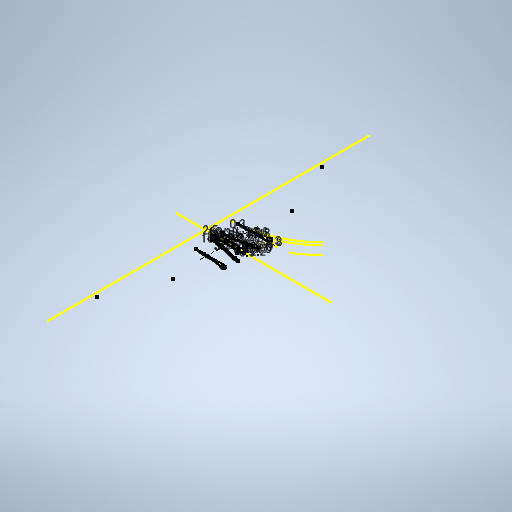
# Autodesk Inventor part: RR_SingleTurnoutLever-ALL
Saved by Autodesk Inventor 2025.1 (Build 291241000, 241)
## iProperties
Created: 2025-03-06
Part Number: RR_SingleTurnoutLever-ALL
Material: 一般
Document SubType Name: Modeling
Designer: kumagai
Density: 1 g/cm^3
Appearance: 既定
Author: kumagai
Autodesk Inventor part; units mm, degrees
ref_plane "YZ Plane" through (0, 0, 0) normal (1, 0, 0) x (0, 1, 0)
ref_plane "XZ Plane" through (0, 0, 0) normal (0, 1, 0) x (-1, 0, 0)
ref_plane "XY Plane" through (0, 0, 0) normal (0, 0, 1) x (1, 0, 0)
derived "RR_ThreeWay.ipt"
sketch "MainSketch" plane through (0, 0, 0) normal (0, 1, 0) x (-1, 0, 0)
  line L0 (0, -344.2613) -> (0, 286.2613)
  line L1 (-272.9287, 0) -> (62.5724, 0)
  line L2 (14.6437, -29) -> (-5, -29)
  line L3 (-5, -49.5106) -> (-5, -5.6416)
  line L4 (-5, -48) -> (0, -48)
  line L5 (-5, -10) -> (0, -10)
  line L6 (-5, -38.3) -> (0, -38.3)
  line L7 (-5, -19.7) -> (0, -19.7)
  line L8 (-5, -46) -> (0, -46)
  line L9 (-5, -35.9) -> (0, -35.9)
  line L10 (-5, -22.1) -> (0, -22.1)
  line L11 (-5, -12) -> (0, -12)
  line L12 (-10, -10) -> (-10, -29)
  line L13 (-225, -48) -> (-225, -29)
  line L14 (-120.9077, -19.7) -> (-225, -19.7)
  arc A0 (-10, -48) -> (-148.5929, -105.4071) centre (-10, -244) ccw
  arc A1 (-10, -46) -> (-150.0071, -103.9929) centre (-10, -244) ccw
  line L15 (-143.2215, -110.7785) -> (-189.5102, -64.4898)
  line L16 (-210, -35.9) -> (-210, -29)
  line L17 (-146.1596, -86.6272) -> (-155.9415, -76.8453)
  arc A2 (-133.8847, -47.8455) -> (-174.0488, -79.9512) centre (-10, -244) ccw
  arc A3 (-139.2229, -48.9168) -> (-175.463, -78.537) centre (-10, -244) ccw
  line L18 (-139.499, -48) -> (-225, -48)
  line L19 (-134.4186, -46) -> (-225, -46)
  arc A4 (-118.9103, -50.6657) -> (-166.907, -87.093) centre (-10, -244) ccw
  arc A5 (-120.0882, -48.5746) -> (-168.6041, -85.3959) centre (-10, -244) ccw
  line L20 (-94.2219, -46) -> (-110.2721, -46)
  arc A6 (-111.9271, -35.5897) -> (-114.1724, -36.7028) centre (-10, -244) ccw
  line L21 (-120.9077, -35.9) -> (-225, -35.9)
  line L22 (-120.9077, -38.3) -> (-225, -38.3)
  arc A7 (-133.8847, -47.8455) -> (-134.4186, -46) centre (-134.4186, -47) ccw
  arc A8 (-139.2229, -48.9168) -> (-139.499, -48) centre (-139.499, -48.5) ccw
  arc A9 (-110.2721, -48.4) -> (-118.9103, -50.6657) centre (-110.2721, -66) ccw
  arc A10 (-110.2721, -46) -> (-120.0882, -48.5746) centre (-110.2721, -66) ccw
  arc A11 (-120.9077, -38.3) -> (-114.1724, -36.7028) centre (-120.9077, -23.3) ccw
  arc A12 (-120.9077, -35.9) -> (-115.25, -34.5584) centre (-120.9077, -23.3) ccw
  arc A13 (-143.5264, -51.2283) -> (-148.5252, -54.7884) centre (-10, -244) ccw
  arc A14 (-112.9815, -33.4337) -> (-115.25, -34.5584) centre (-10, -244) ccw
  line L23 (-120.9077, -22.1) -> (-225, -22.1)
  circle A15 centre (-86.125, -22.2) radius 2.5
  arc A16 (-96.415, -52.9331) -> (-105.3417, -57.2273) centre (-10, -244) ccw
  arc A17 (-96.4922, -49.4759) -> (-95.7188, -53.2122) centre (-89.6121, -50) ccw
  arc A18 (-93.3838, -47.5455) -> (-92.1285, -53.7307) centre (-89.6121, -50) ccw
  arc A19 (-96.1897, -54.5879) -> (-157.1489, -96.8511) centre (-10, -244) ccw
  line L24 (-97.4893, -48.4) -> (-110.2721, -48.4)
  arc A20 (-92.2877, -55.4762) -> (-155.4519, -98.5481) centre (-10, -244) ccw
  arc A21 (-92.2877, -55.4762) -> (-92.1285, -53.7307) centre (-92.6877, -54.5597) ccw
  arc A22 (-93.3838, -47.5455) -> (-94.2219, -46) centre (-94.2219, -47) ccw
  arc A23 (-96.1897, -54.5879) -> (-95.7188, -53.2122) centre (-96.6039, -53.6777) ccw
  arc A24 (-96.4922, -49.4759) -> (-97.4893, -48.4) centre (-97.4893, -49.4) ccw
  circle A25 centre (-89.6121, -50) radius 2.5
  line L25 (-42.4799, -17.7596) -> (-25.8571, -19.9879)
  arc A26 (-25.9153, -20.5847) -> (-85.6348, -24.6515) centre (-40.1446, -252.1479) ccw
  arc A27 (-85.7928, -19.7222) -> (-85.6348, -24.6515) centre (-86.125, -22.2) ccw
  arc A28 (-25.9153, -20.5847) -> (-25.8571, -19.9879) centre (-25.8969, -20.2853) ccw
  arc A29 (-42.4799, -17.7596) -> (-76.3848, -20.5664) centre (-40.1446, -252.1479) ccw
  line L26 (-85.7928, -19.7222) -> (-79.2595, -20.598)
  arc A30 (-79.2595, -20.598) -> (-76.3848, -20.5664) centre (-77.9308, -10.6866) ccw
  circle A31 centre (-89.6121, -50) radius 4
  line L27 (-89.754, -46.0025) -> (-25.5965, -43.7259)
  arc A32 (-25.552, -44.3238) -> (-40.8225, -46.6677) centre (-3.1703, -241.0547) ccw
  arc A33 (-25.552, -44.3238) -> (-25.5965, -43.7259) centre (-25.5859, -44.0257) ccw
  arc A34 (-74.4895, -48.1141) -> (-87.9633, -53.6443) centre (-3.1703, -241.0547) ccw
  line L28 (-72.9332, -47.8071) -> (-40.8225, -46.6677)
  arc A35 (-72.9332, -47.8071) -> (-74.4895, -48.1141) centre (-72.7559, -52.804) ccw
  arc A36 (-44.0479, -18.9806) -> (-84.6326, -23.2308) centre (-40.1446, -252.1479) ccw
  arc A37 (-27.9859, -39.0878) -> (-44.4613, -41.2072) centre (-10, -244) ccw
  line L29 (-31.1334, -19.7) -> (-47.6548, -19.7)
  arc A38 (-10, -22.1) -> (-22.0271, -22.4262) centre (-10, -244) ccw
  arc A39 (-44.7432, -24.8368) -> (-62.9678, -28.5145) centre (-10, -244) ccw
  arc A40 (-10, -19.7) -> (-22.1572, -20.0297) centre (-10, -244) ccw
  arc A41 (-45.119, -22.4664) -> (-72.2793, -28.5197) centre (-10, -244) ccw
  arc A42 (-25.457, -23.6967) -> (-43.178, -22.3501) centre (-51.8841, -254.1867) ccw
  line L30 (-24.9, -22.9254) -> (-24.9, -23.2)
  arc A43 (-25.457, -23.6967) -> (-24.9, -23.2) centre (-25.4, -23.2) ccw
  arc A44 (-22.1572, -20.0297) -> (-24.9, -22.9254) centre (-22, -22.9254) ccw
  arc A45 (-43.178, -22.3501) -> (-45.119, -22.4664) centre (-43.5532, -32.343) ccw
  arc A46 (-25.7303, -26.0811) -> (-43.268, -24.7484) centre (-51.8841, -254.1867) ccw
  arc A47 (-22.0271, -22.4262) -> (-22.5, -22.9254) centre (-22, -22.9254) ccw
  line L31 (-22.5, -22.9254) -> (-22.5, -23.2)
  arc A48 (-25.7303, -26.0811) -> (-22.5, -23.2) centre (-25.4, -23.2) ccw
  arc A49 (-43.268, -24.7484) -> (-44.7432, -24.8368) centre (-43.5532, -32.343) ccw
  line L32 (-55.2, -53.283) -> (-55.2, -10)
  line L33 (-40.8, -50.4351) -> (-40.8, -10)
  line L34 (-48, 3.552) -> (-48, 5.2256)
  line L35 (-59, -61.5) -> (-37, -61.5)
  line L36 (-40.8, -10) -> (-40.8, -7.4996)
  line L37 (-55.2, -10) -> (-55.2, -7.4996)
  line L38 (-48, -61.9179) -> (-48, -64.1825)
  line L39 (-37, -61.5) -> (-37, -70.5)
  line L40 (-40, -73.5) -> (-42, -73.5)
  line L41 (-42, -73.5) -> (-40, -62)
  line L42 (-40, -62) -> (-56, -62)
  line L43 (-56, -62) -> (-54, -73.5)
  line L44 (-54, -73.5) -> (-56, -73.5)
  line L45 (-59, -70.5) -> (-59, -58.1371)
  arc A50 (-40, -73.5) -> (-37, -70.5) centre (-40, -70.5) ccw
  arc A51 (-59, -70.5) -> (-56, -73.5) centre (-56, -70.5) ccw
  line L46 (-37, -61.5) -> (-37, -49.8686)
  line L47 (-40.8, -50.4351) -> (-40.8, -62)
  line L48 (-55.2, -53.283) -> (-55.2, -62)
  arc A52 (-34.3731, -49.5213) -> (-37, -52.498) centre (-34, -52.498) ccw
  arc A53 (-59, -58.1371) -> (-62.8083, -55.2481) centre (-62, -58.1371) ccw
  line L49 (-10, -29) -> (-225, -29)
  arc A54 (-151.7465, 120.5538) -> (-11.4945, 29.8813) centre (-10, 186) ccw
  arc A55 (-22.0271, -35.5738) -> (-10, -35.9) centre (-10, 186) ccw
  arc A56 (-22.1572, -37.9703) -> (-10, -38.3) centre (-10, 186) ccw
  arc A57 (-43.268, -33.2516) -> (-25.7303, -31.9189) centre (-51.8841, 196.1867) ccw
  arc A58 (-43.178, -35.6499) -> (-25.457, -34.3033) centre (-51.8841, 196.1867) ccw
  arc A59 (-62.9678, -29.4855) -> (-44.7432, -33.1632) centre (-10, 186) ccw
  arc A60 (-72.2793, -29.4803) -> (-45.119, -35.5336) centre (-10, 186) ccw
  arc A61 (-45.119, -35.5336) -> (-43.178, -35.6499) centre (-43.5532, -25.657) ccw
  arc A62 (-44.7432, -33.1632) -> (-43.268, -33.2516) centre (-43.5532, -25.657) ccw
  arc A63 (-22.5, -35.0746) -> (-22.0271, -35.5738) centre (-22, -35.0746) ccw
  arc A64 (-24.9, -35.0746) -> (-22.1572, -37.9703) centre (-22, -35.0746) ccw
  line L50 (-24.9, -35.0746) -> (-24.9, -34.8)
  line L51 (-22.5, -35.0746) -> (-22.5, -34.8)
  arc A65 (-24.9, -34.8) -> (-25.457, -34.3033) centre (-25.4, -34.8) ccw
  arc A66 (-22.5, -34.8) -> (-25.7303, -31.9189) centre (-25.4, -34.8) ccw
  arc A67 (-62.9678, -28.5145) -> (-63.3485, -29) centre (-62.8485, -29) ccw
  arc A68 (-72.2793, -28.5197) -> (-72.6405, -29) centre (-72.1405, -29) ccw
  arc A69 (-108.1902, -15.666) -> (-89.3785, -23.7845) centre (-10, 186) ccw
  arc A70 (-91.0057, 5.3288) -> (-16.6975, -11.8867) centre (-10, 186) ccw
  arc A71 (-122.8924, 131.193) -> (-43.8763, 65.1658) centre (-10, 186) ccw
  arc A72 (-148.5252, -3.2116) -> (-143.5264, -6.7717) centre (-10, 186) ccw
  circle A73 centre (-86.125, -35.8) radius 2.5
  arc A74 (-85.7286, -33.3316) -> (-25.8975, -35.1189) centre (-48.9436, 195.7336) ccw
  line L52 (-25.8166, -35.7131) -> (-42.3424, -38.5735)
  arc A75 (-25.8166, -35.7131) -> (-25.8975, -35.1189) centre (-25.8677, -35.4174) ccw
  line L53 (-85.6986, -38.2634) -> (-79.2034, -37.1391)
  arc A76 (-76.3296, -37.0611) -> (-79.2034, -37.1391) centre (-77.4979, -46.9926) ccw
  arc A77 (-76.3296, -37.0611) -> (-42.3424, -38.5735) centre (-48.9436, 195.7336) ccw
  arc A78 (-49.1227, -37.4664) -> (-46.0444, -37.4484) centre (-48.9436, 195.7336) ccw
  line L54 (-86.4807, -38.2746) -> (-94.1197, -37.1765)
  arc A79 (-94.2268, -36.2144) -> (-94.1197, -37.1765) centre (-94.0486, -36.6816) ccw
  line L55 (-87.0159, -33.4641) -> (-94.2268, -36.2144)
  line L56 (-76.4926, -34.8148) -> (-77.6457, -34.6296)
  arc A80 (-96.055, -36.8647) -> (-107.6082, -42.0517) centre (-10, -244) ccw
  circle A81 centre (-89.6121, -8) radius 4
  line L57 (-89.6178, -12) -> (-25.42, -12.0915)
  arc A82 (-88.0883, -4.3016) -> (-74.4341, -9.37) centre (-9.7235, 185.8863) ccw
  arc A83 (-74.4341, -9.37) -> (-72.8683, -9.6239) centre (-72.8611, -4.6239) ccw
  line L58 (-72.8683, -9.6239) -> (-40.7373, -9.6697)
  arc A84 (-40.7373, -9.6697) -> (-25.3959, -11.4925) centre (-9.7235, 185.8863) ccw
  arc A85 (-25.42, -12.0915) -> (-25.3959, -11.4925) centre (-25.4196, -11.7915) ccw
  line L59 (-41.4, -73.5) -> (-41.4, -70.05)
  line L60 (-54.6, -73.5) -> (-54.6, -70.05)
  line L61 (-21.7393, -64.7371) -> (-21.7393, -55.7371)
  line L62 (-51.6, 5.7033) -> (-51.6, 3.6437)
  line L63 (-44.4, 6.6538) -> (-44.4, 3.6437)
  line L64 (-44.4, -63.9796) -> (-44.4, -61.3243)
  line L65 (-51.6, -63.5159) -> (-51.6, -61.3243)
  arc A86 (-106.8215, -31.0506) -> (-105.9722, -29) centre (-108.8722, -29) ccw
  arc A87 (-111.9271, -35.5897) -> (-109.9456, -34.1747) centre (-115.1782, -28.9421) ccw
  line L66 (-109.9456, -34.1747) -> (-106.8215, -31.0506)
  arc A88 (-112.9815, -33.4337) -> (-111.6427, -32.4776) centre (-115.1782, -28.9421) ccw
  arc A89 (-108.5186, -29.3536) -> (-108.3722, -29) centre (-108.8722, -29) ccw
  line L67 (-111.6427, -32.4776) -> (-108.5186, -29.3536)
  arc A90 (-63.3485, -29) -> (-62.9678, -29.4855) centre (-62.8485, -29) ccw
  arc A91 (-72.6405, -29) -> (-72.2793, -29.4803) centre (-72.1405, -29) ccw
  line L68 (-210, -29) -> (-210, -22.1)
  line L69 (-225, -29) -> (-225, -10)
  line L70 (-10, -29) -> (-10, -48)
  line L71 (-22.0231, -12) -> (-39.3668, -12)
  line L72 (-157.1489, -96.8511) -> (-146.5423, -86.2445)
  point P0 (0, 0)
  point P1 (-90.8602, -19.7)
  point P2 (-94.9346, -22.1)
  point P3 (-96.3241, -48.4)
  point P4 (-87.5506, -46)
  point P5 (-162.028, -91.972)
  point P6 (-44.0258, -45.5806)
  point P7 (-48, -2.9806)
  point P8 (-48, -61.5806)
  point P9 (-37, -73.5)
  point P10 (-59, -73.5)
  point P11 (-51.2642, -37.4549)
  point P12 (-51.1178, -10.8549)
  point P13 (-103.3722, -29)
  point P14 (-48, -53.4549)
sketch "LeverSketch" plane through (0, 0, 0) normal (0, 1, 0) x (-1, 0, 0)
  circle A0 centre (-89.6121, -50) radius 4
  circle A1 centre (-86.125, -22.2) radius 2.5
  arc A2 (-26.6638, -12.5992) -> (-85.3134, -24.5646) centre (-10, -244) ccw
  arc A3 (-26.6638, -12.5992) -> (-26.6853, -12) centre (-26.6853, -12.3) ccw
  arc A4 (-43.4568, -12) -> (-76.6882, -19.2867) centre (-10, -244) ccw
  line L0 (-43.4568, -12) -> (-26.6853, -12)
  line L1 (-86.125, -19.7) -> (-79.5332, -19.7)
  arc A5 (-52.0572, -14.6238) -> (-62.7445, -16.8431) centre (-10, -244) ccw
  arc A6 (-79.5332, -19.7) -> (-76.6882, -19.2867) centre (-79.5332, -9.7) ccw
  line L2 (-89.6121, -46) -> (-25.4143, -46)
  line L3 (-59.4552, -48.4) -> (-40.735, -48.4)
  arc A7 (-25.391, -46.5991) -> (-40.735, -48.4) centre (-10, -244) ccw
  arc A8 (-25.391, -46.5991) -> (-25.4143, -46) centre (-25.4143, -46.3) ccw
  line L4 (0, -353.824) -> (0, 343.6373) projected
  line L5 (-272.9287, 0) -> (62.5724, 0) projected
  circle A9 centre (-86.125, 22.2) radius 2.5
  arc A10 (-85.3134, 24.5646) -> (-26.6638, 12.5992) centre (-10, 244) ccw
  arc A11 (-26.6853, 12) -> (-26.6638, 12.5992) centre (-26.6853, 12.3) ccw
  arc A12 (-76.6882, 19.2867) -> (-43.4568, 12) centre (-10, 244) ccw
  line L6 (-43.4568, 12) -> (-26.6853, 12)
  line L7 (-86.125, 19.7) -> (-79.5332, 19.7)
  arc A13 (-76.6882, 19.2867) -> (-79.5332, 19.7) centre (-79.5332, 9.7) ccw
  circle A14 centre (-89.6121, 50) radius 4
  line L8 (-89.6121, 46) -> (-25.4143, 46)
  line L9 (-59.4552, 48.4) -> (-40.735, 48.4)
  arc A15 (-88.1761, 53.7333) -> (-59.4552, 48.4) centre (-59.4552, 128.4) ccw
  arc A16 (-40.735, 48.4) -> (-25.391, 46.5991) centre (-10, 244) ccw
  arc A17 (-25.4143, 46) -> (-25.391, 46.5991) centre (-25.4143, 46.3) ccw
  circle A18 centre (-86.125, -22.2) radius 1.1
  circle A19 centre (-89.6121, -50) radius 1.1
  circle A20 centre (-86.125, 22.2) radius 1.1
  circle A21 centre (-89.6121, 50) radius 1.1
  circle A22 centre (-89.6121, -50) radius 2.4
  circle A23 centre (-86.125, -22.2) radius 2.4
  circle A24 centre (-89.6121, -50) radius 1.65
  circle A25 centre (-86.125, -22.2) radius 1.65
  circle A26 centre (-52.0572, -14.6238) radius 1.6
  circle A27 centre (-51.1138, -47.2) radius 1.6
  circle A28 centre (-52.0572, -14.6238) radius 1.8
  circle A29 centre (-51.1138, -47.2) radius 1.8
  circle A30 centre (-52.0572, 14.6238) radius 1.65
  circle A31 centre (-52.0572, 14.6238) radius 1.85
  circle A32 centre (-51.1138, 47.2) radius 1.65
  circle A33 centre (-51.1138, 47.2) radius 1.85
  line L10 (-60, -5.0418) -> (-60, -4.3264)
  line L11 (-33.7, -3.5) -> (-86.7, -3.5)
  line L12 (-87.2, -3) -> (-87.2, 3)
  line L13 (-86.7, 3.5) -> (-34.7, 3.5)
  arc A34 (-48.1, -1) -> (-45.3, -1) centre (-46.7, -1) ccw
  arc A35 (-45.3, 1) -> (-48.1, 1) centre (-46.7, 1) ccw
  line L14 (-45.3, -1) -> (-45.3, 1)
  line L15 (-48.1, -1) -> (-48.1, 1)
  arc A36 (-74.7, -1) -> (-71.9, -1) centre (-73.3, -1) ccw
  arc A37 (-71.9, 1) -> (-74.7, 1) centre (-73.3, 1) ccw
  line L16 (-74.7, -1) -> (-74.7, 1)
  line L17 (-71.9, -1) -> (-71.9, 1)
  circle A38 centre (-21.2, 3.6) radius 1.6
  arc A39 (-86.7, 3.5) -> (-87.2, 3) centre (-86.7, 3) ccw
  arc A40 (-87.2, -3) -> (-86.7, -3.5) centre (-86.7, -3) ccw
  arc A41 (-59.4552, -48.4) -> (-88.1761, -53.7333) centre (-59.4552, -128.4) ccw
  arc A42 (-10, -46) -> (-150.0071, -103.9929) centre (-10, -244) ccw projected
  arc A43 (-92.2877, -55.4762) -> (-155.4519, -98.5481) centre (-10, -244) ccw projected
  line L18 (-94.2219, -46) -> (-110.2721, -46) projected
  arc A44 (-133.8847, -47.8455) -> (-174.0488, -79.9512) centre (-10, -244) ccw projected
  line L19 (-5, -12) -> (0, -12) projected
  circle A45 centre (-43.8978, -47.2) radius 1.6
  circle A46 centre (-43.8978, -47.2) radius 1.8
  circle A47 centre (-44.8487, -13.4186) radius 1.6
  circle A48 centre (-44.8487, -13.4186) radius 1.8
  circle A49 centre (-43.8978, 47.2) radius 1.6
  circle A50 centre (-43.8978, 47.2) radius 1.8
  circle A51 centre (-44.8487, 13.4186) radius 1.8
  circle A52 centre (-44.8487, 13.4186) radius 1.6
  line L20 (-34.7, 3.5) -> (-34.7, 6.1)
  line L21 (-33.7, 7.1) -> (-20.7, 7.1)
  line L22 (-32.7, -2.5) -> (-32.7, 0.1)
  line L23 (-32.7, 0.1) -> (-20.7, 0.1)
  line L24 (-18.2, 2.6) -> (-18.2, 4.6)
  arc A53 (-20.7, 0.1) -> (-18.2, 2.6) centre (-20.7, 2.6) ccw
  arc A54 (-18.2, 4.6) -> (-20.7, 7.1) centre (-20.7, 4.6) ccw
  arc A55 (-33.7, -3.5) -> (-32.7, -2.5) centre (-33.7, -2.5) ccw
  arc A56 (-33.7, 7.1) -> (-34.7, 6.1) centre (-33.7, 6.1) ccw
  line L25 (-86.6044, -24.6536) -> (-94.1787, -23.1735)
  line L26 (-86.8975, -19.8224) -> (-94.2374, -22.2072)
  arc A57 (-94.2374, -22.2072) -> (-94.1787, -23.1735) centre (-94.0828, -22.6827) ccw
  line L27 (-81.8555, -23.3778) -> (-80.5261, -22.9215)
  line L28 (-86.6044, 24.6536) -> (-94.1787, 23.1735)
  line L29 (-86.8975, 19.8224) -> (-94.2374, 22.2072)
  arc A58 (-94.1787, 23.1735) -> (-94.2374, 22.2072) centre (-94.0828, 22.6827) ccw
  point P0 (0, 0)
  point P1 (-78.0652, -19.7)
  point P2 (-50.0555, -46)
  point P3 (-52.1721, -46)
  point P4 (-52.1721, -48.4)
  point P5 (-50.0555, -48.4)
  point P6 (-51.2296, -13.2545)
  point P7 (-53.3168, -13.6372)
  point P8 (-52.8786, -15.9969)
  point P9 (-50.8021, -15.6161)
  point P10 (-52.4555, -46)
  point P11 (-52.4555, -48.4)
  point P12 (-49.7722, -48.4)
  point P13 (-49.7722, -46)
  point P14 (-53.596, -13.6899)
  point P15 (-53.1563, -16.0493)
  point P16 (-50.5239, -15.5666)
  point P17 (-50.9499, -13.2047)
  point P18 (-49.9813, 48.4)
  point P19 (-52.2463, 48.4)
  point P20 (-52.2463, 46)
  point P21 (-49.9813, 46)
  point P22 (-50.7293, 15.6031)
  point P23 (-52.9513, 16.0106)
  point P24 (-53.3899, 13.651)
  point P25 (-51.1564, 13.2414)
  point P26 (-49.7058, 48.4)
  point P27 (-52.5218, 48.4)
  point P28 (-52.5218, 46)
  point P29 (-49.7058, 46)
  point P30 (-50.4587, 15.555)
  point P31 (-53.2214, 16.0616)
  point P32 (-53.6613, 13.7023)
  point P33 (-50.8844, 13.1931)
  point P34 (-46.7, 2.4)
  point P35 (-46.7, -2.4)
  point P36 (-32.7, -3.5)
  point P37 (-43.9786, -12.0758)
  point P38 (-46.0768, -12.393)
  point P39 (-45.7128, -14.7652)
  point P40 (-43.6253, -14.4497)
  point P41 (-44.9561, -46)
  point P42 (-44.9561, -48.4)
  point P43 (-42.8395, -48.4)
  point P44 (-42.8395, -46)
  point P45 (-45.2394, -46)
  point P46 (-45.2394, -48.4)
  point P47 (-42.5562, -48.4)
  point P48 (-42.5562, -46)
  point P49 (-46.3575, -12.4368)
  point P50 (-45.992, -14.8089)
  point P51 (-43.3457, -14.4089)
  point P52 (-43.6975, -12.0348)
  point P53 (-42.8395, 48.4)
  point P54 (-44.9561, 48.4)
  point P55 (-44.9561, 46)
  point P56 (-42.8395, 46)
  point P57 (-43.6253, 14.4497)
  point P58 (-45.7128, 14.7652)
  point P59 (-46.0768, 12.393)
  point P60 (-43.9786, 12.0758)
  point P61 (-45.2394, 48.4)
  point P62 (-45.2394, 46)
  point P63 (-42.5562, 46)
  point P64 (-42.5562, 48.4)
  point P65 (-43.6975, 12.0348)
  point P66 (-43.3457, 14.4089)
  point P67 (-45.992, 14.8089)
  point P68 (-46.3575, 12.4368)
  dimension "d1" = 8
  dimension "d2" = 5
  dimension "d3" = 0.3
  dimension "d5" = 1.2
  dimension "d24" = 2.4
  dimension "d25" = 10
  dimension "d31" = 2.4
  dimension "d61" = 0.3
  dimension "d64" = 1.2
  dimension "d71" = 2.2
  dimension "d72" = 4.8
  dimension "d81" = 3.3
  dimension "d84" = 3.2
  dimension "d85" = 3.6
  dimension "d90" = 3.3
  dimension "d91" = 3.7
  dimension "d102" = 60
  dimension "d118" = 2.8
  dimension "d119" = 26.6
  dimension "d120" = 4.8
  dimension "d121" = 7
  dimension "d122" = 1.1
  dimension "d124" = 3.2
  dimension "d130" = 80
  dimension "d132" = 38.6
  dimension "d133" = 45.8
  dimension "d134" = 34.9
  dimension "d135" = 42.2
  dimension "d144" = 13.9
  dimension "d145" = 0.5
  dimension "d146" = 3.6
  dimension "d147" = 12
  dimension "d148" = 0.1
  dimension "d149" = 7
  dimension "d152" = 3
  dimension "d153" = 2.5
  dimension "d154" = 1
  dimension "d155" = 14.5
  dimension "d156" = 16.5
  dimension "d157" = 25.5
  dimension "d158" = 30
  dimension "d159" = 0.5
  dimension "d160" = 18
  constraints: 69 point on circle, 56 centre point, 53 end point, 34 symmetric about line, 33 tangent, 26 coincident, 17 equal radius, 6 vertical, 3 horizontal, 3 point on line, 1 collinear, 1 horizontal alignment, 1 parallel, 19 other
  measures "d1" diameter of A0
  measures "d2" diameter of A1
  measures "d3" radius of A3
  measures "d5" radial gap between concentric circles of A4 A5
  measures "d24" radial gap between concentric circles of A4 A2
  measures "d25" radius of A6
  measures "d31" distance between parallel lines of L2 L3
  measures "d61" radius of A8
  measures "d64" distance from line of L2 point (-51.114, -47.2)
  measures "d71" diameter of A18
  measures "d72" diameter of A22
  measures "d81" diameter of A24
  measures "d84" diameter of A26
  measures "d85" diameter of A28
  measures "d90" diameter of A30
  measures "d91" diameter of A31
  measures "d102" distance between parallel lines of L4 L10
  measures "d118" distance between parallel lines of L15 L14
  measures "d119" distance of A36.centre A34.centre
  measures "d120" distance of point (-46.7, 2.4) point (-46.7, -2.4)
  measures "d121" distance between parallel lines of L13 L11
  measures "d122" distance from line of L11 point (-46.7, -2.4)
  measures "d124" diameter of A38
  measures "d130" radius of A41
  measures "d132" distance of point (-51.114, -47.2) point (-89.612, -50)
  measures "d133" distance of A45.centre point (-89.612, -50)
  measures "d134" distance of point (-52.057, -14.624) point (-86.125, -22.2)
  measures "d135" distance of A47.centre point (-86.125, -22.2)
  measures "d144" distance from line of A36.centre L12
  measures "d145" radius of A40
  measures "d146" distance from line of L5 A38.centre
  measures "d147" distance from line of A34.centre L20
  measures "d148" distance between parallel lines of L5 L23
  measures "d149" distance between parallel lines of L21 L23
  measures "d152" distance from line of L24 A38.centre
  measures "d153" radius of A53
  measures "d154" radius of A55
  measures "d155" distance between parallel lines of L24 L22
  measures "d156" distance between parallel lines of L24 L20
  measures "d157" horizontal distance of A38.centre A34.centre
  measures "d158" angle of L27 L25
  measures "d159" radius of A57
  measures "d160" angle of L1 L26
extrude "LeverBody" add sketch "LeverSketch" against normal blind 2.8 contours A0 | A0 L2 A29 L3 A41 | L2 A27 L3 A29 | L2 A27 L3 | A29 L3 A27 L2 | L2 A46 L3 A29 | L2 A45 L3 A46 | L2 A45 L3 | A46 L3 A45 L2 | L2 A8 A7 L3 A46 | A1 | A1 L1 A6 A4 A28 A2 | A1 L25 A57 L26 | A28 A5 A26 A2 | A26 A4 A2 | A28 A4 A26 A5 | A28 A4 A48 A2 | A2 A26 A4 A28 | A48 A4 A47 A2 | A47 A4 A2 | A48 A4 L0 A3 A2 | A2 A47 A4 A48 | A9 | A9 A10 A31 A12 A13 L7 | A9 L29 A58 L28 | A10 A30 A12 A31 | A10 A30 A12 | A31 A12 A30 A10 | A10 A51 A12 A31 | A10 A52 A12 A51 | A10 A52 A12 | A51 A12 A52 A10 | A10 A11 L6 A12 A51 | A14 | A14 A15 L9 A33 L8 | A33 L9 A32 L8 | A32 L9 L8 | A33 L9 A50 L8 | L8 A32 L9 A33 | A50 L9 A49 L8 | A49 L9 L8 | A50 L9 A16 A17 L8 | L8 A49 L9 A50 | A22 | A23 | A24 | A25
extrude "Boss" add sketch "LeverSketch" along normal blind 2.8 contours A22 | A23 | A24 | A25
chamfer "ScrewDish" distance 1 angle 45 2 edges at (87.225, -2.8, 22.2) (90.7121, -2.8, 50)
extrude "InsertHole" cut sketch "LeverSketch" along normal blind 3.4 from surface at -2.8 contours A24 | A25
chamfer "InsertChamfer" distance 0.4 angle 45 2 edges at (91.2621, -2.8, -50) (87.775, -2.8, -22.2)
extrude "PinP1" add sketch "LeverSketch" along normal blind 2.8 contours L2 A27 L3 | A26 A4 A2
extrude "PinP2" add sketch "LeverSketch" along normal blind 2.8 contours L2 A45 L3 | A47 A4 A2
extrude "PinH1" add sketch "LeverSketch" along normal blind 0.4 from surface at 2.8 contours L2 A27 L3 A29 | L2 A27 L3 | A29 L3 A27 L2 | A28 A5 A26 A2 | A26 A4 A2 | A28 A4 A26 A5 | A2 A26 A4 A28
extrude "PinH2" add sketch "LeverSketch" along normal blind 0.4 from surface at 2.8 contours L2 A45 L3 A46 | L2 A45 L3 | A46 L3 A45 L2 | A48 A4 A47 A2 | A47 A4 A2 | A2 A47 A4 A48
extrude "SlotP1" cut sketch "LeverSketch" against normal blind 0.4 contours A10 A30 A12 | A32 L9 L8
extrude "SlotP2" cut sketch "LeverSketch" against normal blind 0.4 contours A10 A52 A12 | A49 L9 L8
extrude "SlotH1" cut sketch "LeverSketch" against normal blind 0.4 from surface at -0.4 contours A10 A30 A12 A31 | A10 A30 A12 | A31 A12 A30 A10 | A33 L9 A32 L8 | A32 L9 L8 | L8 A32 L9 A33
extrude "SlotH2" cut sketch "LeverSketch" against normal blind 0.4 from surface at -0.4 contours A10 A52 A12 A51 | A10 A52 A12 | A51 A12 A52 A10 | A50 L9 A49 L8 | A49 L9 L8 | L8 A49 L9 A50
extrude "SlidePlate" add sketch "LeverSketch" along normal blind 2 from surface at -2.8 contours L12 A39 L13 L20 A56 L21 A54 L24 A53 L23 L22 L5 L14 A35 L15 L17 A37 L16 | L5 L16 A36 L17 L15 A34 L14 L22 A55 L11 A40 L12
mirror "No2Mirror" [suppressed]
